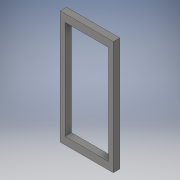
# Autodesk Inventor part: 20_Cube_Insert_Sample_clamp
Saved by Autodesk Inventor 2019.4 (Build 234330000, 330)
## iProperties
Created: 2019-08-09
Part Number: 20_Cube_Insert_Sample_clamp
Material: Generic
Document SubType Name: Modeling
Designer: marsikovabarbora
Density: 1 g/cm^3
Appearance: Default
Author: marsikovabarbora
Autodesk Inventor part; units mm, degrees
ref_plane "YZ Plane" through (0, 0, 0) normal (1, 0, 0) x (0, 1, 0)
ref_plane "XZ Plane" through (0, 0, 0) normal (0, 1, 0) x (-1, 0, 0)
ref_plane "XY Plane" through (0, 0, 0) normal (0, 0, 1) x (1, 0, 0)
sketch "Sketch1" plane through (0, 0, 0) normal (0, 0, 1) x (1, 0, 0)
  line L0 (-17.5, 0) -> (17.5, 0) construction
  line L1 (0, -37.52) -> (0, 37.52) construction
  line L2 (-12.5, 26.8) -> (12.5, 26.8)
  line L3 (12.5, 26.8) -> (12.5, -26.8)
  line L4 (12.5, -26.8) -> (-12.5, -26.8)
  line L5 (-12.5, -26.8) -> (-12.5, 26.8)
  line L6 (-10.25, 23.3) -> (10.25, 23.3)
  line L7 (10.25, 23.3) -> (10.25, -23.3)
  line L8 (10.25, -23.3) -> (-10.25, -23.3)
  line L9 (-10.25, -23.3) -> (-10.25, 23.3)
  point P0 (0, 0)
  dimension "d0" = 20.5
  dimension "d1" = 25
  dimension "d3" = 46.6
  dimension "d8" = 3.5
  dimension "d9" = 3.5
  dimension "d10" = 53.6
  constraints: 16 end point, 4 parallel, 2 horizontal, 2 perpendicular, 4 other
  measures "d0" distance of L6.start L6.end
  measures "d1" distance of L2.start L2.end
  measures "d3" distance of L6.end L7.end
  measures "d8" distance between parallel lines of L2 L6
  measures "d9" distance between parallel lines of L4 L8
  measures "d10" distance between parallel lines of L4 L2
extrude "Extrusion1" add sketch "Sketch1" along normal blind 3
body "Solid1"
